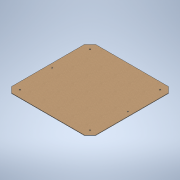
# Autodesk Inventor part: fundo falso
Saved by Autodesk Inventor 2022 (Build 260153000, 153)
## iProperties
Created: 2022-02-16
Part Number: fundo falso
Material: MDF - Chapa de fibra de média densidade
Document SubType Name: Modeling
Designer: mathe
Density: 0.8 g/cm^3
Appearance: Papelão - Corrugado
Author: mathe
Autodesk Inventor part; units mm, degrees
ref_plane "YZ Plane" through (0, 0, 0) normal (1, 0, 0) x (0, 1, 0)
ref_plane "XZ Plane" through (0, 0, 0) normal (0, 1, 0) x (-1, 0, 0)
ref_plane "XY Plane" through (0, 0, 0) normal (0, 0, 1) x (1, 0, 0)
sketch "Esboço1" plane through (0, 0, 0) normal (0, 1, 0) x (-1, 0, 0)
  line L0 (0, 0) -> (600, 0)
  line L1 (600, 0) -> (600, -600)
  line L2 (600, -600) -> (0, -600)
  line L3 (0, -600) -> (0, 0)
  constraints: 8 end point, 2 parallel, 1 horizontal, 1 perpendicular
extrude "Extrusão1" add sketch "Esboço1" along normal blind 3
sketch "Esboço2" plane through (0, 3, 0) normal (0, 1, 0) x (1, 0, 0)
  point P0 (0, 0)
  point P1 (-50, 50)
  point P2 (-550, 50)
  point P3 (-50, 550)
  point P4 (-550, 550)
hole "Furo1" at (-50, 3, -50) at (-550, 3, -50) at (-50, 3, -550) at (-550, 3, -550) direction (0, -1, 0) diameter 8 end through all
sketch "Esboço3" plane through (0, 3, 0) normal (0, 1, 0) x (1, 0, 0)
  line L0 (0, 0) -> (0, 600) projected
  line L1 (-600, 600) -> (-600, 0) projected
  point P0 (-29.956, 300)
  point P1 (-570.044, 300)
  dimension "d18" = 29.956
  dimension "d19" = 29.956
  measures "d18" distance from line of L0 point (-29.956, 300)
  measures "d19" distance from line of L1 point (-570.044, 300)
hole "Furo2" at (-29.956, 3, -300) at (-570.044, 3, -300) direction (0, -1, 0) diameter 8 end through all
sketch "Esboço4" plane through (0, 3, 0) normal (0, 1, 0) x (1, 0, 0)
  line L0 (-600, 0) -> (0, 0) projected
  line L1 (0, 0) -> (0, 40)
  line L2 (0, 0) -> (0, 600) projected
  line L3 (0, 40) -> (-40, 0)
  line L4 (-40, 0) -> (0, 0)
  line L5 (0, 600) -> (-40, 600)
  line L6 (0, 600) -> (-600, 600) projected
  line L7 (-40, 600) -> (0, 560)
  line L8 (0, 600) -> (0, 560)
  line L9 (-600, 600) -> (-600, 0) projected
  line L10 (-600, 600) -> (-600, 560)
  line L11 (-600, 560) -> (-560, 600)
  line L12 (-560, 600) -> (-600, 600)
  line L13 (-600, 0) -> (-600, 40)
  line L14 (-600, 40) -> (-560, 0)
  line L15 (-560, 0) -> (-600, 0)
  dimension "d20" = 40
  dimension "d21" = 45
  dimension "d22" = 40
  constraints: 24 end point, 8 point on line, 2 collinear, 1 perpendicular
  measures "d20" distance of L0.end L1.end
  measures "d21" angle of L3 L1
  measures "d22" distance of L2.end L5.end
extrude "Extrusão2" cut sketch "Esboço4" against normal through all contours L9 L14 L0 | L3 L1 L0 | L9 L6 L11 | L7 L5 L2
